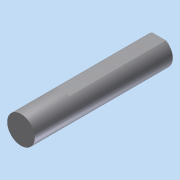
# Autodesk Inventor part: Motoraxle
Saved by Autodesk Inventor 2012 (Build 160160000, 160)
## iProperties
Created: 2011-10-28
Part Number: Motoraxle
Material: Default
Document SubType Name: Modeling
Designer: Kyle
Density: 1 g/cm^3
Author: Kyle
Autodesk Inventor part; units mm, degrees
ref_plane "YZ Plane" through (0, 0, 0) normal (1, 0, 0) x (0, 1, 0)
ref_plane "XZ Plane" through (0, 0, 0) normal (0, 1, 0) x (-1, 0, 0)
ref_plane "XY Plane" through (0, 0, 0) normal (0, 0, 1) x (1, 0, 0)
sketch "Sketch1" plane through (0, 0, 0) normal (0, 0, 1) x (1, 0, 0)
  arc A0 (-1.5875, 2.7496) -> (1.5875, 2.7496) centre (0, 0) ccw
  line L0 (-1.5875, 2.7496) -> (1.5875, 2.7496)
  dimension "d0" = 6.35
  dimension "d1" = 3.175
  constraints: 2 end point, 2 point on circle, 1 centre point, 1 coincident, 1 horizontal
  measures "d0" diameter of A0
  measures "d1" distance of L0.start L0.end
extrude "Extrusion1" add sketch "Sketch1" along normal blind 31.75
sketch "Sketch2" plane through (0, 0, 31.75) normal (0, 0, 1) x (1, 0, 0)
  line L0 (-1.5875, 2.7496) -> (1.5875, 2.7496) projected
  arc A0 (-1.5875, 2.7496) -> (1.5875, 2.7496) centre (0, 0) ccw projected
  arc A1 (1.5875, 2.7496) -> (-1.5875, 2.7496) centre (0, 0) ccw
  line L1 (-1.5875, 2.7496) -> (1.5875, 2.7496)
  constraints: 2 end point, 2 point on circle, 1 centre point, 1 coincident, 1 collinear, 1 concentric
extrude "Extrusion2" add sketch "Sketch2" against normal blind 9.525 contours A1 L0
body "Solid1"
